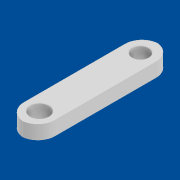
# Autodesk Inventor part: GRIPPER1
Saved by Autodesk Inventor 2020 (Build 240168000, 168)
## iProperties
Created: 2022-02-12
Part Number: GRIPPER1
Material: Generic
Document SubType Name: Modeling
Designer: niladri
Density: 1 g/cm^3
Appearance: Default
Author: niladri
Autodesk Inventor part; units mm, degrees
ref_plane "YZ Plane" through (0, 0, 0) normal (1, 0, 0) x (0, 1, 0)
ref_plane "XZ Plane" through (0, 0, 0) normal (0, 1, 0) x (-1, 0, 0)
ref_plane "XY Plane" through (0, 0, 0) normal (0, 0, 1) x (1, 0, 0)
sketch "Sketch1" plane through (0, 0, 0) normal (0, 1, 0) x (-1, 0, 0)
  line L0 (6.3007, 16.0107) -> (6.8999, 16.0107)
  line L1 (3.7249, 12.8357) -> (3.7249, -5.8651)
  line L2 (6.8999, -9.0401) -> (6.3007, -9.0401)
  line L3 (9.4757, -5.8651) -> (9.4757, 12.8357)
  arc A0 (9.4757, 12.8357) -> (6.3007, 16.0107) centre (6.3007, 12.8357) ccw
  arc A1 (6.3007, -9.0401) -> (9.4757, -5.8651) centre (6.3007, -5.8651) ccw
  arc A2 (3.7249, -5.8651) -> (6.8999, -9.0401) centre (6.8999, -5.8651) ccw
  arc A3 (6.8999, 16.0107) -> (3.7249, 12.8357) centre (6.8999, 12.8357) ccw
  circle A4 centre (6.6003, 12.8357) radius 1.745
  circle A5 centre (6.6003, -5.8651) radius 1.5248
  point P0 (0, 0)
  point P1 (6.6003, 15.9965)
  point P2 (6.6003, -9.0259)
  dimension "d0" = 3.175
  constraints: 8 end point, 8 point on circle, 8 tangent, 6 centre point, 3 equal radius, 2 parallel, 1 horizontal, 1 perpendicular
  measures "d0" radius of A0
extrude "Extrusion1" add sketch "Sketch1" along normal blind 2.54 contours A0 L3 A1 A2 L1 A3
body "Solid1"
